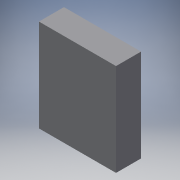
# Autodesk Inventor part: TCS3472
Saved by Autodesk Inventor 2016 (Build 200138000, 138)
## iProperties
Created: 2016-01-30
Part Number: TCS3472
Material: Generic
Document SubType Name: Modeling
Designer: jferner
Density: 1 g/cm^3
Appearance: Default
TCS3472_x: 2.000 mm
TCS3472_y: 2.400 mm
TCS3472_z: 0.650 mm
Author: jferner
Autodesk Inventor part; units mm, degrees
ref_plane "YZ Plane" through (0, 0, 0) normal (1, 0, 0) x (0, 1, 0)
ref_plane "XZ Plane" through (0, 0, 0) normal (0, 1, 0) x (-1, 0, 0)
ref_plane "XY Plane" through (0, 0, 0) normal (0, 0, 1) x (1, 0, 0)
sketch "Sketch1" plane through (0, 0, 0) normal (0, 1, 0) x (-1, 0, 0)
  line L0 (0, 0) -> (-2, 0)
  line L1 (-2, 0) -> (-2, -2.4)
  line L2 (-2, -2.4) -> (0, -2.4)
  line L3 (0, -2.4) -> (0, 0)
  dimension "TCS3472_x" = 2
  dimension "TCS3472_y" = 2.4
  constraints: 8 end point, 2 parallel, 1 horizontal, 1 perpendicular
  measures "TCS3472_x" distance of L1.end L2.end
  measures "TCS3472_y" distance of L0.end L1.end
extrude "Extrusion1" add sketch "Sketch1" along normal blind 0.65
body "Solid1"
